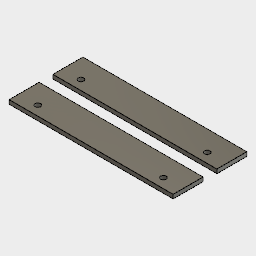
Box Secure v3 (Autodesk Fusion 360 design; units mm, degrees)
Autodesk Fusion 360 part; units mm, degrees
sketch "Sketch1" plane through (0, 0, 0) normal (0, 1, 0) x (1, 0, 0)
  line L0 (0, 0) -> (120, 0)
  line L1 (120, 0) -> (120, 22)
  line L2 (120, 22) -> (0, 22)
  line L3 (0, 22) -> (0, 0)
  line L4 (0, 0) -> (22, 22)
  line L5 (120, 0) -> (98, 22)
  circle A0 centre (13.6029, 7) radius 2
  circle A1 centre (105.9289, 7) radius 2
  dimension "d1" = 22
  dimension "d2" = 120
  dimension "d4" = 45
  dimension "d5" = 45
  dimension "d7" = 4
  dimension "d8" = 4
  dimension "d10" = 7
  dimension "d11" = 5
  dimension "d14" = 7
  constraint horizontal L0
  constraint vertical L1
  constraint horizontal L2
  constraint vertical L3
  constraint coincident L2
  measures "d4" angle of L0 L4
  measures "d5" angle of L1 L5
  measures "d7" diameter of A0
  measures "d8" diameter of A1
  measures "d10" distance of L0
  measures "d11" distance of L5
  measures "d14" distance of L0
extrude "Extrude1" add sketch "Sketch1" along normal blind 3 makes body 1
sketch "Sketch2" plane through (0, 0, 0) normal (0, 1, 0) x (1, 0, 0)
  line L0 (0, -10) -> (120, -10)
  line L1 (120, -10) -> (120, -32)
  line L2 (120, -32) -> (0, -32)
  line L3 (0, -32) -> (0, -10)
  line L4 (0, -32) -> (22, -10)
  line L5 (120, -32) -> (98, -10)
  circle A0 centre (14.0711, -25) radius 2
  circle A1 centre (105.9289, -25) radius 2
  dimension "d19" = 22
  dimension "d20" = 45
  dimension "d21" = 45
  dimension "d22" = 4
  dimension "d23" = 4
  dimension "d24" = 7
  dimension "d25" = 5
  dimension "d26" = 7
  dimension "d27" = 5
  constraint horizontal L0
  constraint vertical L1
  constraint horizontal L2
  constraint vertical L3
  constraint coincident L0
  constraint midpoint L4
  measures "d20" angle of L2 L4
  measures "d21" angle of L2 L5
  measures "d22" diameter of A0
  measures "d23" diameter of A1
  measures "d24" distance of L2
  measures "d25" distance of L4
  measures "d26" distance of L2
  measures "d27" distance of L5
extrude "Extrude2" add sketch "Sketch2" along normal blind 3 separate body makes body 2
